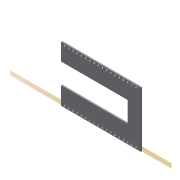
# Autodesk Inventor part: Flat Roof panel
Saved by Autodesk Inventor 2018 (Build 220112000, 112)
## iProperties
Created: 2019-01-04
Part Number: Flat Roof panel
Material: Generic
Document SubType Name: Modeling
Designer: ball
Density: 1 g/cm^3
Appearance: Default
Author: ball
Autodesk Inventor part; units mm, degrees
ref_plane "YZ Plane" through (0, 0, 0) normal (1, 0, 0) x (0, 1, 0)
ref_plane "XZ Plane" through (0, 0, 0) normal (0, 1, 0) x (-1, 0, 0)
ref_plane "XY Plane" through (0, 0, 0) normal (0, 0, 1) x (1, 0, 0)
ref_plane "Work Plane1" through (0, 0, 0) normal (0, 0, 1) x (1, 0, 0)
sketch "Sketch1" plane through (0, 0, 0) normal (0, 0, 1) x (1, 0, 0)
  line L0 (272, -4) -> (-8, -4) construction
  line L1 (230, 0) -> (230, -3.492) construction
  line L2 (272, 102.8084) -> (-8, 102.8084) construction
  line L3 (62, 0) -> (62, -4) construction
  line L4 (78, 0) -> (78, -3.492) construction
  circle A0 centre (220, 0) radius 2 construction
  circle A1 centre (164, 0) radius 2 construction
  circle A2 centre (148, 0) radius 2 construction
  circle A3 centre (140, 0) radius 2 construction
  circle A4 centre (132, 0) radius 2 construction
  circle A5 centre (124, 0) radius 2 construction
  circle A6 centre (116, 0) radius 2 construction
  circle A7 centre (108, 0) radius 2 construction
  circle A8 centre (100, 0) radius 2 construction
  circle A9 centre (92, 0) radius 2 construction
  circle A10 centre (84, 0) radius 2 construction
  circle A11 centre (84, 98.8084) radius 2 construction
  circle A12 centre (92, 98.8084) radius 2 construction
  circle A13 centre (100, 98.8084) radius 2 construction
  circle A14 centre (108, 98.8084) radius 2 construction
  circle A15 centre (116, 98.8084) radius 2 construction
  circle A16 centre (124, 98.8084) radius 2 construction
  circle A17 centre (132, 98.8084) radius 2 construction
  circle A18 centre (140, 98.8084) radius 2 construction
  circle A19 centre (148, 98.8084) radius 2 construction
  circle A20 centre (156, 98.8084) radius 2 construction
  circle A21 centre (164, 98.8084) radius 2 construction
  circle A22 centre (172, 98.8084) radius 2 construction
  circle A23 centre (180, 98.8084) radius 2 construction
  circle A24 centre (188, 98.8084) radius 2 construction
  circle A25 centre (196, 98.8084) radius 2 construction
  circle A26 centre (204, 98.8084) radius 2 construction
  circle A27 centre (212, 98.8084) radius 2 construction
  circle A28 centre (220, 98.8084) radius 2 construction
  circle A29 centre (212, 0) radius 2 construction
  circle A30 centre (204, 0) radius 2 construction
  circle A31 centre (196, 0) radius 2 construction
  circle A32 centre (188, 0) radius 2 construction
  circle A33 centre (180, 0) radius 2 construction
  circle A34 centre (172, 0) radius 2 construction
  circle A35 centre (156, 0) radius 2 construction
  circle A36 centre (220, 0) radius 2.2479
  circle A37 centre (211.999, 0) radius 2.2479
  circle A38 centre (203.998, 0) radius 2.2479
  circle A39 centre (195.997, 0) radius 2.2479
  circle A40 centre (187.996, 0) radius 2.2479
  circle A41 centre (179.995, 0) radius 2.2479
  circle A42 centre (171.994, 0) radius 2.2479
  circle A43 centre (163.993, 0) radius 2.2479
  circle A44 centre (155.992, 0) radius 2.2479
  circle A45 centre (147.991, 0) radius 2.2479
  circle A46 centre (139.99, 0) radius 2.2479
  circle A47 centre (131.989, 0) radius 2.2479
  circle A48 centre (123.988, 0) radius 2.2479
  circle A49 centre (115.987, 0) radius 2.2479
  circle A50 centre (107.986, 0) radius 2.2479
  circle A51 centre (99.985, 0) radius 2.2479
  circle A52 centre (91.984, 0) radius 2.2479
  circle A53 centre (83.983, 0) radius 2.2479
  circle A54 centre (220, 98.8084) radius 2.2479
  circle A55 centre (211.999, 98.8084) radius 2.2479
  circle A56 centre (203.998, 98.8084) radius 2.2479
  circle A57 centre (195.997, 98.8084) radius 2.2479
  circle A58 centre (187.996, 98.8084) radius 2.2479
  circle A59 centre (179.995, 98.8084) radius 2.2479
  circle A60 centre (171.994, 98.8084) radius 2.2479
  circle A61 centre (163.993, 98.8084) radius 2.2479
  circle A62 centre (155.992, 98.8084) radius 2.2479
  circle A63 centre (147.991, 98.8084) radius 2.2479
  circle A64 centre (139.99, 98.8084) radius 2.2479
  circle A65 centre (131.989, 98.8084) radius 2.2479
  circle A66 centre (123.988, 98.8084) radius 2.2479
  circle A67 centre (115.987, 98.8084) radius 2.2479
  circle A68 centre (107.986, 98.8084) radius 2.2479
  circle A69 centre (99.985, 98.8084) radius 2.2479
  circle A70 centre (91.984, 98.8084) radius 2.2479
  circle A71 centre (83.983, 98.8084) radius 2.2479
  line L5 (78, 30.29) -> (205, 30.29)
  line L6 (205, 30.29) -> (205, 69.6341)
  line L7 (205, 69.6341) -> (78, 69.6341)
  line L8 (78, -3.492) -> (78, 30.29)
  line L9 (78, 69.6341) -> (78, 102.3004)
  line L10 (78, -3.492) -> (230, -3.492)
  line L11 (230, 102.3004) -> (78, 102.3004)
  line L12 (230, -3.492) -> (230, 102.3004)
  point P0 (0, 0)
  point P1 (-8, -4)
  dimension "d0" = 4.4958
  dimension "d3" = 8.001
  dimension "d8" = 4.4958
  dimension "d11" = 8.001
  constraints: 72 centre point, 24 end point, 17 equal radius, 17 horizontal alignment, 4 vertical, 3 horizontal, 2 coincident, 2 perpendicular, 1 parallel, 118 other
  measures "d0" diameter of A36
  measures "d3" distance of A36.centre A37.centre
  measures "d8" diameter of A54
  measures "d11" distance of A54.centre A55.centre
extrude "Extrusion1" add sketch "Sketch1" along normal blind 2.54
body "Solid1"
